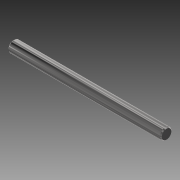
# Autodesk Inventor part: 80mm shaft
Saved by Autodesk Inventor 2015 (Build 190159000, 159)
## iProperties
Created: 2013-07-07
Part Number: 80mm shaft
Material: Generic
Document SubType Name: Modeling
Designer: mhgreen
Density: 1 g/cm^3
Appearance: Default
Catalog Web Link: http://www.sdp-si.com/eStore/Catalog/PartNumber/S40PX0MHG6M-080
Description: 6 (-.004/-.012) Dia; 80mm Long; 416 Stainless Steel Shaft
Vendor: SDP/SI
Author: mhgreen
Autodesk Inventor part; units mm, degrees
ref_plane "YZ Plane" through (0, 0, 0) normal (1, 0, 0) x (0, 1, 0)
ref_plane "XZ Plane" through (0, 0, 0) normal (0, 1, 0) x (-1, 0, 0)
ref_plane "XY Plane" through (0, 0, 0) normal (0, 0, 1) x (1, 0, 0)
sketch "Sketch1" plane through (0, 0, 0) normal (1, 0, 0) x (0, 1, 0)
  circle A0 centre (0, 0) radius 3
  dimension "d0" = 6
  constraints: 1 centre point, 1 coincident
  measures "d0" diameter of A0
extrude "Extrusion1" add sketch "Sketch1" along normal blind 80
chamfer "Chamfer1" distance 0.5 angle 45 2 edges at (80, -3, 0) (0, -3, 0)
body "Solid1"
